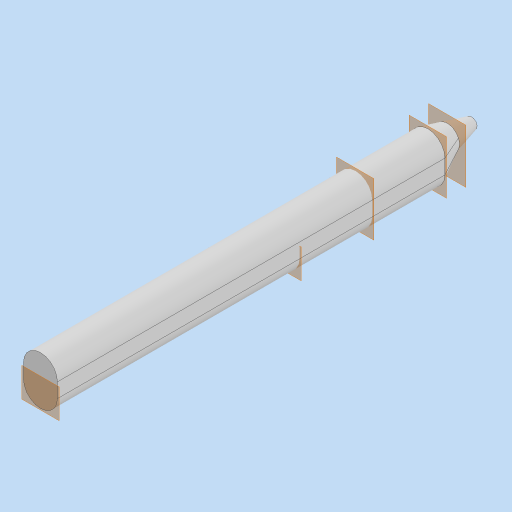
# Autodesk Inventor part: Form_test
Saved by Autodesk Inventor 2024 (Build 280153000, 153)
## iProperties
Created: 2025-03-21
Part Number: Form_test
Material: Generic
Document SubType Name: Modeling
Designer: XxPan
Density: 1 g/cm^3
Appearance: Default
Author: XxPan
Autodesk Inventor part; units mm, degrees
ref_plane "YZ Plane" through (0, 0, 0) normal (1, 0, 0) x (0, 1, 0)
ref_plane "XZ Plane" through (0, 0, 0) normal (0, 1, 0) x (-1, 0, 0)
sketch "Sketch4" plane through (0, 0, 0) normal (0, 0, -1) x (-1, 0, 0)
  circle A0 centre (0, 0) radius 5
  dimension "d17" = 10
  constraints: 1 centre point, 1 coincident
  measures "d17" diameter of A0
ref_plane "Work Plane3" through (0, 0, 8) normal (0, 0, 1) x (1, 0, 0)
sketch "Sketch1" plane through (0, 0, 8) normal (0, 0, 1) x (1, 0, 0)
  line L0 (0, 0) -> (0, -6) construction
  line L1 (-7, 0) -> (-7, -6)
  line L2 (7, -6) -> (7, 0)
  arc A0 (7, 0) -> (-7, 0) centre (0, 0) ccw
  arc A1 (-7, -6) -> (7, -6) centre (0, -6) ccw
  point P0 (0, -3)
  dimension "d0" = 6
  dimension "d1" = 14
  constraints: 8 end point, 4 point on circle, 4 tangent, 2 centre point, 1 midpoint, 1 parallel, 1 vertical
  measures "d0" distance of L0.start L0.end
  measures "d1" diameter of A1
extrude "Extrusion1" add sketch "Sketch1" along normal blind 30
ref_plane "Work Plane1" through (0, 0, 68) normal (0, 0, 1) x (1, 0, 0)
ref_plane "Work Plane2" through (0, 0, 168) normal (0, 0, 1) x (1, 0, 0)
sketch "Sketch2" plane through (0, 0, 68) normal (0, 0, 1) x (1, 0, 0)
  arc A0 (-7, -6) -> (7, -6) centre (0, -6) ccw projected
  line L0 (7, -6) -> (7, 0) projected
  arc A1 (7, 0) -> (-7, 0) centre (0, 0) ccw projected
  line L1 (-7, 0) -> (-7, -6) projected
extrude "Extrusion2" add sketch "Sketch2" along normal up to surface (100 mm away)
loft "Loft1" add section 1 edges at (0, -13, 38) (7, -3, 38) (0, 7, 38) (-7, -3, 38) section 2 edges at (7, -3, 68) (0, -13, 68) (-7, -3, 68) (0, 7, 68)
ref_plane "Work Plane4" through (0, 0, 38) normal (0, 0, 1) x (1, 0, 0)
loft "Loft2" add profiles "Sketch4" section 1 edges at (0, -13, 8) (-7, -3, 8) (0, 7, 8) (7, -3, 8)
sketch "Sketch5" plane through (0, 0, 0) normal (0, 0, -1) x (-1, 0, 0)
  arc A0 (-4.5957, -1.9696) -> (4.5957, -1.9696) centre (0, 0) ccw projected
  arc A1 (4.5957, -1.9696) -> (4.5957, 1.9696) centre (0, 0) ccw projected
  arc A2 (4.5957, 1.9696) -> (-4.5957, 1.9696) centre (0, 0) ccw projected
  arc A3 (-4.5957, 1.9696) -> (-4.5957, -1.9696) centre (0, 0) ccw projected
extrude "Extrusion4" add sketch "Sketch5" along normal blind 10 draft -15
body "Solid1"
